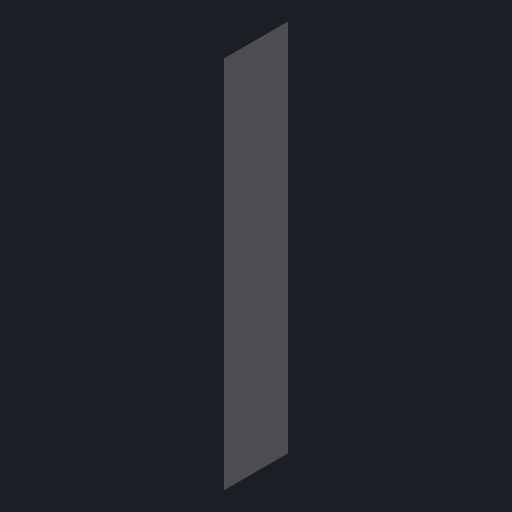
# Autodesk Inventor part: CARCASA_ALUM_1_FLAT
Saved by Autodesk Inventor 2024.3 (Build 283343000, 343)
## iProperties
Created: 2024-05-15
Part Number: CARCASA_ALUM_1_FLAT
Material: Steel, Mild, Welded
Document SubType Name: Modeling
Designer: Niler
Density: 7.85 g/cm^3
Appearance: Weld - Steel Mild
Author: Niler
Autodesk Inventor part; units mm, degrees
ref_plane "YZ Plane" through (0, 0, 0) normal (1, 0, 0) x (0, 1, 0)
ref_plane "XZ Plane" through (0, 0, 0) normal (0, 1, 0) x (-1, 0, 0)
ref_plane "XY Plane" through (0, 0, 0) normal (0, 0, 1) x (1, 0, 0)
sketch "Sketch1" plane through (0, 0, 0) normal (1, 0, 0) x (0, 1, 0)
  line L0 (0, 0) -> (5285.3133, 0)
  line L1 (0, -450) -> (0, 0)
  line L2 (5285.3133, -450) -> (0, -450)
  line L3 (5285.3133, 0) -> (5285.3133, -450)
  line L4 (2642.6566, 0) -> (2642.6566, -450)
  constraints: 10 end point, 2 horizontal, 2 midpoint, 2 vertical, 1 coincident, 5 other
extrude "Extrusion1" add sketch "Sketch1" along normal blind 1.5 contours L0 L4 L2 L1
body "Solid1"
